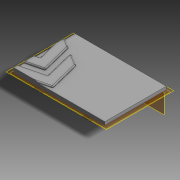
# Autodesk Inventor part: Deckel
Saved by Autodesk Inventor 2014 (Build 180170000, 170)
## iProperties
Created: 2016-07-15
Part Number: Deckel
Material: Generisch
Document SubType Name: Modeling
Designer: cem
Density: 1 g/cm^3
Appearance: Vorgabe
Author: cem
Autodesk Inventor part; units mm, degrees
ref_plane "YZ Plane" through (0, 0, 0) normal (1, 0, 0) x (0, 1, 0)
ref_plane "XZ Plane" through (0, 0, 0) normal (0, 1, 0) x (-1, 0, 0)
ref_plane "XY Plane" through (0, 0, 0) normal (0, 0, 1) x (1, 0, 0)
ref_plane "Arbeitsebene1" through (0, 0, 0) normal (0, 0, 1) x (1, 0, 0)
sketch "Skizze1" plane through (0, 0, 0) normal (0, 0, 1) x (1, 0, 0)
  line L0 (20.75, 13.75) -> (20.75, -13.75) projected
  line L1 (20.75, -13.75) -> (-20.75, -13.75) projected
  line L2 (-20.75, -13.75) -> (-20.75, 13.75) projected
  line L3 (-20.75, 13.75) -> (20.75, 13.75) projected
  line L4 (21.5, 14.5) -> (21.5, -14.5) projected
  line L5 (-21.5, 14.5) -> (21.5, 14.5) projected
  line L6 (-21.5, -14.5) -> (-21.5, 14.5) projected
  line L7 (21.5, -14.5) -> (-21.5, -14.5) projected
  line L8 (-21.5, 14.5) -> (21.5, 14.5)
  line L9 (21.5, 14.5) -> (21.5, -14.5)
  line L10 (21.5, -14.5) -> (-21.5, -14.5)
  line L11 (-21.5, -14.5) -> (-21.5, 14.5)
  point P0 (0, 0)
  dimension "d0" = 0
  constraints: 8 end point, 3 other
  measures "d0" distance between parallel lines of L11 L6
extrude "Deckel" add sketch "Skizze1" along normal blind 1.5 contours L0 L1 L2 L3 | L4 L7 L6 L5
ref_plane "Arbeitsebene2" through (0, 0, -0.5) normal (0, 0, 1) x (1, 0, 0)
sketch "Skizze2" plane through (0, 0, -0.5) normal (0, 0, 1) x (1, 0, 0)
  line L0 (-20, 13) -> (-20, -13) projected
  line L1 (20, 13) -> (-20, 13) projected
  line L2 (20, -13) -> (20, 13) projected
  line L3 (-20, -13) -> (20, -13) projected
  line L4 (20.75, -13.75) -> (-20.75, -13.75) projected
  line L5 (20.75, 13.75) -> (20.75, -13.75) projected
  line L6 (-20.75, 13.75) -> (20.75, 13.75) projected
  line L7 (-20.75, -13.75) -> (-20.75, 13.75) projected
  point P0 (0, 0)
extrude "Führung" add sketch "Skizze2" along normal up to next contours L1 L2 L3 L0 | L4 L7 L6 L5
ref_plane "Arbeitsebene4" through (20, 13, -8.8) normal (0, -1, 0) x (-1, 0, 0)
ref_plane "Arbeitsebene5" through (20, 13, -8.8) normal (0, -1, 0) x (-1, 0, 0)
ref_plane "Arbeitsebene6" through (20, 13, -8.8) normal (0, -1, 0) x (-1, 0, 0)
sketch "Skizze10" plane through (20, 13, -8.8) normal (0, -1, 0) x (-1, 0, 0)
  line L0 (7, -4.8) -> (10, -4.8) projected
  line L1 (10, -4.8) -> (10, -6.8) projected
  line L2 (10, -6.8) -> (7, -6.8) projected
  line L3 (7, -6.8) -> (7, -4.8) projected
  line L4 (30, -4.8) -> (33, -4.8) projected
  line L5 (33, -4.8) -> (33, -6.8) projected
  line L6 (33, -6.8) -> (30, -6.8) projected
  line L7 (30, -6.8) -> (30, -4.8) projected
  line L8 (19, -7) -> (19, -3) projected
  line L9 (19, -3) -> (27.5, -3) projected
  line L10 (27.5, -3) -> (27.5, -7) projected
  line L11 (27.5, -7) -> (19, -7) projected
  line L12 (0, -8.3) -> (40, -8.3) projected
  line L13 (40, 0) -> (40, -8.3) projected
  line L14 (0, 0) -> (40, 0) projected
  line L15 (0, 0) -> (0, -8.3) projected
  line L16 (31.5, -4.444) -> (31.5, -7.3143) construction
  line L17 (32.8, -8.3) -> (30.2, -8.3)
  line L18 (30.2, -8.3) -> (30.2, -5)
  line L19 (30.2, -5) -> (32.8, -5)
  line L20 (32.8, -5) -> (32.8, -8.3)
  line L21 (8.5, -7.3143) -> (8.5, -4.2721) construction
  line L22 (9.8, -8.3) -> (7.2, -8.3)
  line L23 (7.2, -8.3) -> (7.2, -5)
  line L24 (7.2, -5) -> (9.8, -5)
  line L25 (9.8, -5) -> (9.8, -8.3)
  point P0 (20, -8.8)
  point P1 (31.5, -6.8)
  point P2 (8.5, -6.8)
  dimension "d22" = 0.2
  dimension "d23" = 0.2
  dimension "d24" = 0.2
  dimension "d25" = 0.2
  constraints: 20 end point, 6 parallel, 4 point on line, 2 horizontal, 2 midpoint, 2 perpendicular, 2 other
  measures "d22" distance between parallel lines of L5 L20
  measures "d23" distance between parallel lines of L4 L19
  measures "d24" distance between parallel lines of L25 L1
  measures "d25" distance between parallel lines of L0 L24
extrude "Extrusion6" add sketch "Skizze10" along normal blind 1.5 contours L23 L24 L25 L2 | L2 L25 L12 L23 | L18 L6 L20 L12 | L18 L19 L20 L6
sketch "Skizze11" plane through (20, 13, -8.8) normal (0, 1, 0) x (1, 0, 0)
  line L0 (-30.2, -5) -> (-30.2, -8.3) projected
  line L1 (-32.8, -5) -> (-30.2, -5) projected
  line L2 (-9.8, -8.3) -> (-9.8, -5) projected
  line L3 (-7.2, -8.3) -> (-9.8, -8.3) projected
  line L4 (-7.2, -5) -> (-7.2, -8.3) projected
  line L5 (-9.8, -5) -> (-7.2, -5) projected
  line L6 (-33, -6.8) -> (-30, -6.8) projected
  line L7 (-10, -6.8) -> (-7, -6.8) projected
  line L8 (-10, -4.8) -> (-10, -6.8) projected
  line L9 (-7, -4.8) -> (-10, -4.8) projected
  line L10 (-7, -6.8) -> (-7, -4.8) projected
  line L11 (-30, -6.8) -> (-30, -4.8) projected
  line L12 (-30, -4.8) -> (-33, -4.8) projected
  line L13 (-33, -4.8) -> (-33, -6.8) projected
  line L14 (-32.8, -5) -> (-30.2, -5)
  line L15 (-30.2, -5) -> (-30.2, -6.6)
  line L16 (-30.2, -6.6) -> (-32.8, -6.6)
  line L17 (-32.8, -6.6) -> (-32.8, -5)
  line L18 (-9.8, -5) -> (-7.2, -5)
  line L19 (-7.2, -5) -> (-7.2, -6.6)
  line L20 (-7.2, -6.6) -> (-9.8, -6.6)
  line L21 (-9.8, -6.6) -> (-9.8, -5)
  point P0 (-20, -8.8)
  dimension "d28" = 0.2
  dimension "d29" = 0.2
  constraints: 16 end point, 4 parallel, 2 horizontal, 2 perpendicular, 2 point on line
  measures "d28" distance between parallel lines of L6 L16
  measures "d29" distance between parallel lines of L7 L20
extrude "Extrusion7" add sketch "Skizze11" along normal blind 0.9 contours L0 L16 L17 L1 | L2 L5 L4 L20
chamfer "Fase3" distance 1.2 angle 45 2 edges at (11.5, 13.9, -3.8) (-11.5, 13.9, -3.8)
mirror "Spiegeln2" about plane through (0, 0, 0) normal (0, 1, 0) of "Extrusion6", "Extrusion7", "Fase3"
sketch "Skizze14" plane through (0, 0, 1.5) normal (0, 0, 1) x (1, 0, 0)
  line L0 (-21.5, 14.5) -> (-21.5, -14.5) projected
  line L1 (-21.5, -14.5) -> (21.5, -14.5) projected
  line L2 (-10.542, -9.4422) -> (-14.181, 5.1097)
  line L3 (-14.181, 5.1097) -> (-8.1173, 1.4721)
  line L4 (-8.1173, 1.4721) -> (-4.4783, -13.0798)
  line L5 (-10.542, -9.4422) -> (-21.5, -12.1824)
  line L6 (-10.1576, -14.5) -> (-4.4783, -13.0798)
  line L7 (-19.6136, -4) -> (-21.5, 3.5436)
  line L8 (-21.5, 9.5005) -> (-17.1889, 6.9143)
  line L9 (-17.1889, 6.9143) -> (-13.5499, -7.6376)
  line L10 (-21.5, -9.6257) -> (-13.5499, -7.6376)
  line L11 (-19.6136, -4) -> (-21.5, -4.4717)
  point P0 (0, 0)
  constraints: 20 end point, 6 point on line, 2 parallel
extrude "Pfeile" add sketch "Skizze14" along normal blind 0.6 contours L8 L9 L10 L0 L11 L7 | L5 L2 L3 L4 L6 L1 L0
fillet "Rundung1" radius 0.5 17 edges at (-19.6136, -4, 1.8) (-20.5568, -0.2282, 2.1) (-19.3445, 8.2074, 2.1) (-17.1889, 6.9143, 1.8) (-15.3694, -0.3617, 2.1) (-13.5499, -7.6376, 1.8) (-17.525, -8.6317, 2.1) (-20.5568, -4.2359, 2.1) (-16.021, -10.8123, 2.1) (-10.542, -9.4422, 1.8) (-12.3615, -2.1662, 2.1) (-14.181, 5.1097, 1.8) (-11.1491, 3.2909, 2.1) (-8.1173, 1.4721, 1.8) (-6.2978, -5.8038, 2.1) (-4.4783, -13.0798, 1.8) (-7.318, -13.7899, 2.1)
